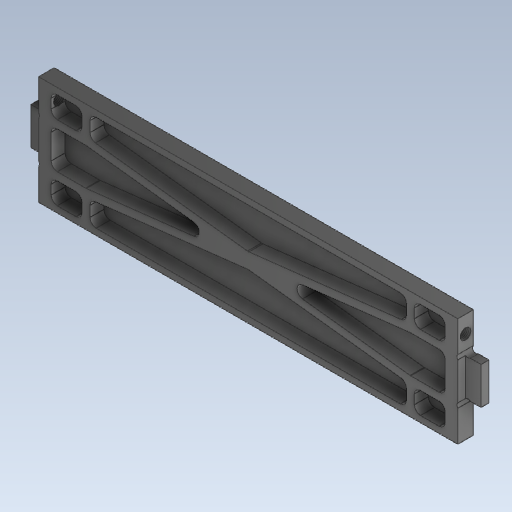
# Autodesk Inventor part: Cockpit_battery_front_frame
Saved by Autodesk Inventor 2020.4 (Build 244396000, 396)
## iProperties
Part Number: Cockpit_battery_front_frame
Material: アセタール樹脂、黒
Document SubType Name: Modeling
Designer: Masato Kubotera
Density: 1.425 g/cm^3
Appearance: 滑らか - 黒
Description: POM T5
Mass: 13.79 g
Surface Area: 149.623 cm^2
Volume: 9.6772 cm^3
Author: Masato Kubotera
Autodesk Inventor part; units mm, degrees
ref_plane "XZ Plane" through (0, 0, 0) normal (0, 1, 0) x (-1, 0, 0)
ref_plane "XY Plane" through (0, 0, 0) normal (0, 0, 1) x (1, 0, 0)
derived "Cockpit_side_frame.ipt"
sketch "スケッチ2" plane through (0, 0, 0) normal (0, 1, 0) x (-1, 0, 0)
  line L0 (-23.5, -22.5) -> (-28.5, -27.5)
  line L1 (-28.5, -27.5) -> (-28.5, -91)
  line L2 (-28.5, -91) -> (-23.5, -96)
  line L3 (-23.5, -96) -> (35.75, -96)
  line L4 (37.75, -98) -> (37.75, -131)
  line L5 (37.75, -131) -> (42.75, -136)
  line L6 (42.75, -136) -> (83.5, -136)
  line L7 (88.5, -131) -> (88.5, -20)
  line L8 (88.5, -20) -> (86, -17.5)
  line L9 (86, -17.5) -> (80.25, -17.5)
  line L10 (80.25, -17.5) -> (80.25, -21.0151)
  line L11 (78.7651, -22.5) -> (73.9849, -22.5)
  line L12 (72.5, -21.0151) -> (72.5, -17.5)
  line L13 (72.5, -17.5) -> (64.5, -17.5)
  line L14 (64.5, -17.5) -> (64.5, -21.0151)
  line L15 (63.0151, -22.5) -> (-23.5, -22.5)
  line L16 (-25.25, -25) -> (-20.25, -25) construction
  line L17 (-20.25, -25) -> (-20.25, -93.5) construction
  line L18 (-20.25, -93.5) -> (-25.25, -93.5) construction
  line L19 (-25.25, -93.5) -> (-25.25, -25) construction
  line L20 (-26, -25) -> (-25.25, -25) construction
  line L21 (-25.25, -93.5) -> (-26, -93.5) construction
  line L22 (-26, -93.5) -> (-26, -25) construction
  line L23 (-20.25, -93.5) -> (80.25, -93.5) construction
  line L24 (-20.25, -88.5) -> (80.25, -88.5) construction
  line L25 (80.25, -22.5) -> (80.25, -90.5) construction
  line L26 (80.25, -90.5) -> (85.25, -90.5) construction
  line L27 (85.25, -90.5) -> (85.25, -22.5) construction
  line L28 (80.25, -88.5) -> (80.25, -93.5) construction
  line L29 (80.25, -91) -> (85.25, -91) construction
  line L30 (85.25, -91) -> (85.25, -133.5) construction
  line L31 (80.25, -91) -> (80.25, -133.5) construction
  line L32 (80.25, -133.5) -> (85.25, -133.5) construction
  line L33 (40.25, -133.5) -> (40.25, -128.5) construction
  line L34 (40.25, -128.5) -> (40.25, -93.5) construction
  line L35 (45.25, -93.5) -> (45.25, -128.5) construction
  line L36 (40.25, -128.5) -> (45.25, -128.5) construction
  line L37 (42.75, -128.5) -> (42.75, -93.5) construction
  line L38 (40.25, -128.5) -> (79.1145, -128.5) construction
  line L39 (79.1145, -128.5) -> (79.1145, -133.5) construction
  line L40 (79.1145, -133.5) -> (40.25, -133.5) construction
  line L41 (40.25, -131) -> (79.1145, -131) construction
  line L42 (82.75, -91) -> (82.75, -133.5) construction
  circle A0 centre (82.75, -131) radius 2
  arc A1 (80.25, -128.5) -> (85.25, -128.5) centre (82.75, -131) ccw construction
  line L43 (80.25, -91) -> (-20.25, -91) construction
  line L44 (42.75, -111) -> (45.25, -111) construction
  line L45 (59.6822, -128.5) -> (59.6822, -131) construction
  line L46 (42.7, -115.5651) -> (42.7, -106.4349)
  line L47 (45.3, -107.05) -> (45.3, -114.95)
  line L48 (45.3, -117.05) -> (42.7, -104.95) construction
  line L49 (42.7, -117.05) -> (45.3, -104.95) construction
  line L50 (55.7322, -128.45) -> (63.6322, -128.45)
  line L51 (64.2473, -131.05) -> (55.1172, -131.05)
  line L52 (53.6322, -128.45) -> (65.7322, -131.05) construction
  line L53 (65.7322, -128.45) -> (53.6322, -131.05) construction
  line L54 (42.75, -105) -> (45.25, -105) construction
  line L55 (42.75, -117) -> (45.25, -117) construction
  arc A2 (44.1849, -104.95) -> (42.7, -106.4349) centre (43.4425, -105.6925) ccw
  arc A3 (45.3, -107.05) -> (45.3, -104.95) centre (45.3, -106) ccw
  arc A4 (42.7, -115.5651) -> (44.1849, -117.05) centre (43.4425, -116.3075) ccw
  arc A5 (45.3, -117.05) -> (45.3, -114.95) centre (45.3, -116) ccw
  line L56 (53.6822, -131) -> (53.6822, -128.5) construction
  line L57 (65.6822, -128.5) -> (65.6822, -131) construction
  arc A6 (53.6322, -129.5651) -> (55.1172, -131.05) centre (54.3747, -130.3075) ccw
  arc A7 (55.7322, -128.45) -> (53.6322, -128.45) centre (54.6822, -128.45) ccw
  arc A8 (64.2473, -131.05) -> (65.7322, -129.5651) centre (64.9898, -130.3075) ccw
  arc A9 (65.7322, -128.45) -> (63.6322, -128.45) centre (64.6822, -128.45) ccw
  line L58 (53.6322, -129.5651) -> (53.6322, -128.45)
  line L59 (65.7322, -128.45) -> (65.7322, -129.5651)
  line L60 (44.1849, -104.95) -> (45.3, -104.95)
  line L61 (45.3, -117.05) -> (44.1849, -117.05)
  circle A10 centre (47.6822, -131) radius 1.6
  line L62 (85.25, -22.5) -> (85.25, -17.5) construction
  line L63 (86, -17.5) -> (86, -90.5) construction
  line L64 (86, -90.5) -> (85.25, -90.5) construction
  line L65 (-18.5, -82.5) -> (-18.5, -61)
  arc A11 (-18.5, -82.5) -> (-16.5, -84.5) centre (-16.5, -82.5) ccw
  line L66 (45.5, -84.5) -> (-16.5, -84.5)
  arc A12 (45.5, -84.5) -> (47.5, -82.5) centre (45.5, -82.5) ccw
  line L67 (47.5, -61) -> (47.5, -82.5)
  arc A13 (47.5, -61) -> (45.5, -59) centre (45.5, -61) ccw
  line L68 (-16.5, -59) -> (45.5, -59)
  arc A14 (-16.5, -59) -> (-18.5, -61) centre (-16.5, -61) ccw
  line L69 (30, -88.5) -> (30, -91) construction
  line L70 (82.75, -22.5) -> (82.75, -90.5) construction
  circle A15 centre (82.75, -34) radius 1.6
  circle A16 centre (82.75, -34) radius 3
  circle A17 centre (82.75, -79) radius 3
  circle A18 centre (82.75, -79) radius 1.6
  line L71 (85.25, -22.5) -> (80.25, -22.5) construction
  arc A19 (85.25, -91) -> (80.25, -91) centre (82.75, -131) ccw construction
  circle A20 centre (47.6822, -131) radius 3
  circle A21 centre (42.75, -99) radius 1.6
  circle A22 centre (42.75, -99) radius 3
  line L72 (5, -88.5) -> (5, -91) construction
  line L73 (55, -88.5) -> (55, -91) construction
  line L74 (53.5651, -91.05) -> (6.4349, -91.05)
  line L75 (4.95, -89.5651) -> (4.95, -88.45)
  line L76 (7.05, -88.45) -> (52.95, -88.45)
  line L77 (55.05, -88.45) -> (55.05, -89.5651)
  line L78 (55.05, -91.05) -> (4.95, -88.45) construction
  line L79 (4.95, -91.05) -> (55.05, -88.45) construction
  arc A23 (7.05, -88.45) -> (4.95, -88.45) centre (6, -88.45) ccw
  arc A24 (4.95, -89.5651) -> (6.4349, -91.05) centre (5.6925, -90.3075) ccw
  arc A25 (53.5651, -91.05) -> (55.05, -89.5651) centre (54.3075, -90.3075) ccw
  arc A26 (55.05, -88.45) -> (52.95, -88.45) centre (54, -88.45) ccw
  line L80 (-20.25, -41) -> (80.25, -41) construction
  line L81 (80.25, -36) -> (-20.25, -36) construction
  line L82 (-20.25, -36) -> (-20.25, -41) construction
  line L83 (-20.25, -38.5) -> (80.25, -38.5) construction
  line L84 (30, -41) -> (30, -36) construction
  line L85 (53.5651, -35.95) -> (6.4349, -35.95)
  line L86 (6.4349, -41.05) -> (53.5651, -41.05)
  line L87 (55.05, -35.95) -> (4.95, -41.05) construction
  line L88 (4.95, -35.95) -> (55.5723, -41.1032) construction
  arc A27 (6.4349, -35.95) -> (4.95, -37.4349) centre (5.6925, -36.6925) ccw
  arc A28 (4.95, -39.5651) -> (6.4349, -41.05) centre (5.6925, -40.3075) ccw
  arc A29 (55.05, -37.4349) -> (53.5651, -35.95) centre (54.3075, -36.6925) ccw
  arc A30 (53.5651, -41.05) -> (55.05, -39.5651) centre (54.3075, -40.3075) ccw
  line L89 (5, -41) -> (5, -36) construction
  line L90 (55, -36) -> (55, -41) construction
  line L91 (4.95, -37.4349) -> (4.95, -39.5651)
  line L92 (55.05, -39.5651) -> (55.05, -37.4349)
  circle A31 centre (-2.5, -38.5) radius 1.6
  circle A32 centre (-2.5, -38.5) radius 3
  circle A33 centre (62.5, -38.5) radius 1.6
  circle A34 centre (62.5, -38.5) radius 3
  line L93 (-25.25, -44.25) -> (-22.75, -44.25) construction
  line L94 (-25.25, -49.25) -> (-26, -49.25) construction
  line L95 (-25.25, -74.25) -> (-22.75, -74.25) construction
  line L96 (-25.25, -69.25) -> (-26, -69.25) construction
  line L97 (-26, -59.25) -> (-25.25, -59.25) construction
  line L98 (-25.25, -59.25) -> (-22.75, -59.25) construction
  line L99 (-22.75, -25) -> (-22.75, -93.5) construction
  arc A35 (63.0151, -22.5) -> (64.5, -21.0151) centre (63.7575, -21.7575) ccw
  arc A36 (72.5, -21.0151) -> (73.9849, -22.5) centre (73.2425, -21.7575) ccw
  line L100 (56.75, -22.5) -> (56.75, -32.5) construction
  line L101 (56.75, -32.5) -> (80.25, -32.5) construction
  line L102 (80.25, -32.5) -> (80.25, -22.5) construction
  line L103 (68.5, -17.5) -> (68.5, -32.5) construction
  line L104 (60.5, -22.5) -> (60.5, -17.5) construction
  line L105 (76.5, -22.5) -> (76.5, -17.5) construction
  line L106 (-22.7, -46.3) -> (-22.7, -72.2)
  line L107 (-25.3, -72.8151) -> (-25.3, -69.564)
  line L108 (-25.3, -44.2) -> (-22.7, -74.3) construction
  line L109 (-22.7, -44.2) -> (-25.3, -74.3) construction
  arc A37 (-22.7, -46.3) -> (-22.7, -44.2) centre (-22.7, -45.25) ccw
  arc A38 (-23.8151, -44.2) -> (-25.3, -45.6849) centre (-24.5575, -44.9425) ccw
  line L110 (-23.8151, -44.2) -> (-22.7, -44.2)
  arc A39 (-25.3, -72.8151) -> (-23.8151, -74.3) centre (-24.5575, -73.5575) ccw
  arc A40 (-22.7, -74.3) -> (-22.7, -72.2) centre (-22.7, -73.25) ccw
  line L111 (-22.7, -74.3) -> (-23.8151, -74.3)
  line L112 (-26.3, -49.9848) -> (-26.3, -68.5152)
  arc A41 (-26.3, -68.5152) -> (-25.3, -69.564) centre (-25.25, -68.5152) ccw
  arc A42 (-25.3, -48.936) -> (-26.3, -49.9848) centre (-25.25, -49.9848) ccw
  line L113 (-25.3, -48.936) -> (-25.3, -45.6849)
  circle A43 centre (-22.75, -36.75) radius 1.6
  circle A44 centre (-22.75, -36.75) radius 3
  circle A45 centre (-22.75, -81.75) radius 1.6
  circle A46 centre (-22.75, -81.75) radius 3
  line L114 (64.5, -22.5) -> (72.5, -22.5)
  line L115 (85.25, -17.5) -> (52.5, -17.5) construction
  line L116 (52.5, -17.5) -> (52.5, -22.5) construction
  circle A47 centre (82.75, -93.5) radius 1.475
  circle A48 centre (82.75, -98.5) radius 1.475
  circle A49 centre (82.75, -103.5) radius 1.475
  line L117 (49.75, -93.5) -> (78.25, -93.5)
  line L118 (80.25, -95.5) -> (80.25, -124)
  line L119 (78.25, -126) -> (49.75, -126)
  line L120 (47.75, -124) -> (47.75, -95.5)
  arc A50 (49.75, -93.5) -> (47.75, -95.5) centre (49.75, -95.5) ccw
  arc A51 (47.75, -124) -> (49.75, -126) centre (49.75, -124) ccw
  arc A52 (78.25, -126) -> (80.25, -124) centre (78.25, -124) ccw
  arc A53 (80.25, -95.5) -> (78.25, -93.5) centre (78.25, -95.5) ccw
  arc A54 (37.75, -98) -> (35.75, -96) centre (35.75, -98) ccw
  circle A55 centre (-13.5, -55) radius 1.75
  circle A56 centre (-13.5, -55) radius 2
  line L121 (74.85, -78.65) -> (65.65, -78.65) construction
  line L122 (65.65, -78.65) -> (65.65, -64.85) construction
  line L123 (65.65, -64.85) -> (74.85, -64.85) construction
  line L124 (74.85, -64.85) -> (74.85, -78.65) construction
  line L125 (74.85, -78.65) -> (65.65, -64.85) construction
  line L126 (65.65, -78.65) -> (74.85, -64.85) construction
  line L127 (64.95, -64.2) -> (75.55, -64.2) construction
  line L128 (75.55, -64.2) -> (75.55, -79.3) construction
  line L129 (75.55, -79.3) -> (64.95, -79.3) construction
  line L130 (64.95, -79.3) -> (64.95, -64.2) construction
  line L131 (64.95, -64.2) -> (75.55, -79.3) construction
  line L132 (75.55, -64.2) -> (64.95, -79.3) construction
  line L133 (66.3849, -64.15) -> (74.1151, -64.15)
  line L134 (75.6, -65.6349) -> (75.6, -77.8651)
  line L135 (75.6, -79.35) -> (64.9, -64.15) construction
  line L136 (64.9, -79.35) -> (75.6, -64.15) construction
  line L137 (74.9, -78.7) -> (65.6, -64.8) construction
  line L138 (65.6, -78.7) -> (74.9, -64.8) construction
  arc A57 (66.3849, -64.15) -> (64.9, -65.6349) centre (65.6425, -64.8925) ccw
  arc A58 (67.0849, -64.8) -> (65.6, -66.2849) centre (66.3425, -65.5425) ccw
  line L139 (64.9, -71.75) -> (75.6, -71.75) construction
  line L140 (70.25, -64.15) -> (70.25, -78.7063) construction
  arc A59 (75.6, -65.6349) -> (74.1151, -64.15) centre (74.8575, -64.8925) ccw
  arc A60 (74.9, -66.2849) -> (73.4151, -64.8) centre (74.1575, -65.5425) ccw
  arc A61 (65.6, -77.2151) -> (67.0849, -78.7) centre (66.3425, -77.9575) ccw
  arc A62 (64.9, -77.8651) -> (66.3849, -79.35) centre (65.6425, -78.6075) ccw
  arc A63 (73.4151, -78.7) -> (74.9, -77.2151) centre (74.1575, -77.9575) ccw
  arc A64 (74.1151, -79.35) -> (75.6, -77.8651) centre (74.8575, -78.6075) ccw
  line L141 (67.0849, -64.8) -> (73.4151, -64.8)
  line L142 (74.9, -66.2849) -> (74.9, -77.2151)
  line L143 (64.9, -77.8651) -> (64.9, -65.6349)
  line L144 (65.6, -77.2151) -> (65.6, -66.2849)
  line L145 (73.4151, -78.7) -> (67.0849, -78.7)
  line L146 (74.1151, -79.35) -> (66.3849, -79.35)
  line L147 (-18.5, -71.75) -> (47.5, -71.75) construction
  line L148 (82.75, -56.5) -> (85.25, -56.5) construction
  line L149 (86, -54) -> (85.25, -54) construction
  line L150 (82.7, -69.45) -> (82.7, -43.55)
  line L151 (85.3057, -71.616) -> (82.7, -41.45) construction
  line L152 (82.7, -71.55) -> (85.3, -41.45) construction
  arc A65 (82.7, -41.45) -> (82.7, -43.55) centre (82.7, -42.5) ccw
  arc A66 (85.3, -42.9349) -> (83.8151, -41.45) centre (84.5575, -42.1925) ccw
  arc A67 (82.7, -69.45) -> (82.7, -71.55) centre (82.7, -70.5) ccw
  arc A68 (83.8151, -71.55) -> (85.3, -70.0651) centre (84.5575, -70.8075) ccw
  line L153 (82.75, -41.5) -> (85.25, -41.5) construction
  line L154 (82.75, -71.5) -> (85.25, -71.5) construction
  arc A69 (86.25, -47.1801) -> (85.3, -46.1348) centre (85.2, -47.1801) ccw
  line L155 (86.25, -47.1801) -> (86.25, -65.8199)
  line L156 (85.25, -46.5) -> (86, -46.5) construction
  line L157 (85.25, -66.5) -> (86, -66.5) construction
  arc A70 (85.3, -66.8652) -> (86.25, -65.8199) centre (85.2, -65.8199) ccw
  line L158 (85.3, -42.9349) -> (85.3, -46.1348)
  line L159 (85.3, -66.8652) -> (85.3, -70.0651)
  line L160 (83.8151, -71.55) -> (82.7, -71.55)
  line L161 (82.7, -41.45) -> (83.8151, -41.45)
  line L162 (83.5, -136) -> (88.5, -131)
  arc A71 (78.7651, -22.5) -> (80.25, -21.0151) centre (79.5075, -21.7575) ccw
  point P0 (0, 0)
  point P1 (-25.7227, -96)
  point P2 (-23.5, -22.5)
  point P3 (44, -111)
  point P4 (59.6822, -129.75)
  point P5 (30, -89.75)
  point P6 (30, -38.5)
  point P7 (4.95, -41.05)
  point P8 (52.5, -22)
  point P9 (-24, -59.25)
  point P10 (70.25, -71.75)
  point P11 (70.25, -71.75)
  point P12 (84, -56.5)
  point P13 (80.25, -22.5)
  dimension "d1" = 45.25
  dimension "d2" = 5
  dimension "d3" = 2.5
  measures "d1" distance from line of point (0, 0) L35
  measures "d2" distance of L35.end L33.end
  measures "d3" distance of L55.start L55.end
ref_plane "作業平面1" through (-45.25, 0, 0) normal (1, 0, 0) x (0, 1, 0)
sketch "スケッチ3" plane through (-45.25, 0, 0) normal (1, 0, 0) x (0, 1, 0)
  line L0 (-135, -93.5) -> (0, -93.5)
  line L1 (0, -128.5) -> (-135, -128.5)
  line L2 (1.4849, -105) -> (5, -105)
  line L3 (5, -105) -> (5, -117)
  arc A0 (0, -103.5151) -> (1.4849, -105) centre (0.7425, -104.2575) ccw
  line L4 (0, -93.5) -> (0, -103.5151)
  line L5 (-134.9908, -111) -> (0, -111) construction
  line L6 (1.4849, -117) -> (5, -117)
  arc A1 (1.4849, -117) -> (0, -118.4849) centre (0.7425, -117.7425) ccw
  line L7 (0, -128.5) -> (0, -118.4849)
  line L8 (0, -105) -> (0, -117)
  line L9 (0, -118.4849) -> (0, -128.5)
  line L10 (-67.5, -93.5) -> (-67.5, -128.5) construction
  line L11 (-136.4849, -105) -> (-140, -105)
  line L12 (-140, -105) -> (-140, -117)
  arc A2 (-136.4849, -105) -> (-135, -103.5151) centre (-135.7425, -104.2575) ccw
  line L13 (-135, -93.5) -> (-135, -103.5151)
  line L14 (-136.4849, -117) -> (-140, -117)
  arc A3 (-135, -118.4849) -> (-136.4849, -117) centre (-135.7425, -117.7425) ccw
  line L15 (-135, -128.5) -> (-135, -118.4849)
  line L16 (-135, -105) -> (-135, -117)
  line L17 (-135, -118.4849) -> (-135, -128.5)
  line L18 (-12, -119.5) -> (-6, -119.5)
  line L19 (-4, -121.5) -> (-4, -124.5)
  line L20 (-6, -126.5) -> (-12, -126.5)
  line L21 (-14, -124.5) -> (-14, -121.5)
  line L22 (-4, -115) -> (-4, -107)
  line L23 (-67.2707, -113.5132) -> (-18.2707, -119.168)
  line L24 (-16.5, -121.1548) -> (-16.5, -124.5)
  line L25 (-18.5, -126.5) -> (-116.5, -126.5)
  line L26 (-6, -117) -> (-15.135, -117)
  line L27 (-15.3643, -116.9868) -> (-50.0251, -112.9868)
  line L28 (-12, -102.5) -> (-6, -102.5)
  line L29 (-4, -100.5) -> (-4, -97.5)
  line L30 (-6, -95.5) -> (-12, -95.5)
  line L31 (-14, -97.5) -> (-14, -100.5)
  line L32 (-67.2707, -108.4868) -> (-18.2707, -102.832)
  line L33 (-16.5, -100.8452) -> (-16.5, -97.5)
  line L34 (-18.5, -95.5) -> (-116.5, -95.5)
  line L35 (-6, -105) -> (-15.135, -105)
  line L36 (-15.3643, -105.0132) -> (-50.0251, -109.0132)
  line L37 (-67.7293, -113.5132) -> (-116.7293, -119.168)
  line L38 (-118.5, -121.1548) -> (-118.5, -124.5)
  line L39 (-118.5, -100.8452) -> (-118.5, -97.5)
  line L40 (-67.7293, -108.4868) -> (-116.7293, -102.832)
  arc A4 (-6, -126.5) -> (-4, -124.5) centre (-6, -124.5) ccw
  arc A5 (-4, -121.5) -> (-6, -119.5) centre (-6, -121.5) ccw
  arc A6 (-12, -119.5) -> (-14, -121.5) centre (-12, -121.5) ccw
  arc A7 (-14, -124.5) -> (-12, -126.5) centre (-12, -124.5) ccw
  arc A8 (-18.5, -126.5) -> (-16.5, -124.5) centre (-18.5, -124.5) ccw
  arc A9 (-16.5, -121.1548) -> (-18.2707, -119.168) centre (-18.5, -121.1548) ccw
  arc A10 (-67.2707, -113.5132) -> (-67.7293, -113.5132) centre (-67.5, -115.5) ccw
  arc A11 (-116.7293, -119.168) -> (-118.5, -121.1548) centre (-116.5, -121.1548) ccw
  arc A12 (-118.5, -124.5) -> (-116.5, -126.5) centre (-116.5, -124.5) ccw
  arc A13 (-118.5, -100.8452) -> (-116.7293, -102.832) centre (-116.5, -100.8452) ccw
  arc A14 (-116.5, -95.5) -> (-118.5, -97.5) centre (-116.5, -97.5) ccw
  arc A15 (-16.5, -97.5) -> (-18.5, -95.5) centre (-18.5, -97.5) ccw
  arc A16 (-18.2707, -102.832) -> (-16.5, -100.8452) centre (-18.5, -100.8452) ccw
  arc A17 (-67.7293, -108.4868) -> (-67.2707, -108.4868) centre (-67.5, -106.5) ccw
  arc A18 (-50.0251, -109.0132) -> (-50.0251, -112.9868) centre (-49.7958, -111) ccw
  arc A19 (-15.135, -105) -> (-15.3643, -105.0132) centre (-15.135, -107) ccw
  arc A20 (-4, -107) -> (-6, -105) centre (-6, -107) ccw
  arc A21 (-6, -117) -> (-4, -115) centre (-6, -115) ccw
  arc A22 (-15.3643, -116.9868) -> (-15.135, -117) centre (-15.135, -115) ccw
  arc A23 (-14, -100.5) -> (-12, -102.5) centre (-12, -100.5) ccw
  arc A24 (-12, -95.5) -> (-14, -97.5) centre (-12, -97.5) ccw
  arc A25 (-4, -97.5) -> (-6, -95.5) centre (-6, -97.5) ccw
  arc A26 (-6, -102.5) -> (-4, -100.5) centre (-6, -100.5) ccw
  line L41 (-123, -119.5) -> (-129, -119.5)
  line L42 (-121, -124.5) -> (-121, -121.5)
  line L43 (-131, -115) -> (-131, -107)
  line L44 (-129, -117) -> (-119.865, -117)
  line L45 (-119.6357, -116.9868) -> (-84.9749, -112.9868)
  line L46 (-123, -102.5) -> (-129, -102.5)
  line L47 (-121, -97.5) -> (-121, -100.5)
  line L48 (-129, -95.5) -> (-123, -95.5)
  line L49 (-131, -100.5) -> (-131, -97.5)
  line L50 (-119.6357, -105.0132) -> (-84.9749, -109.0132)
  line L51 (-129, -105) -> (-119.865, -105)
  arc A27 (-131, -124.5) -> (-129, -126.5) centre (-129, -124.5) ccw
  arc A28 (-129, -119.5) -> (-131, -121.5) centre (-129, -121.5) ccw
  arc A29 (-121, -121.5) -> (-123, -119.5) centre (-123, -121.5) ccw
  arc A30 (-123, -126.5) -> (-121, -124.5) centre (-123, -124.5) ccw
  arc A31 (-84.9749, -112.9868) -> (-84.9749, -109.0132) centre (-85.2042, -111) ccw
  arc A32 (-119.6357, -105.0132) -> (-119.865, -105) centre (-119.865, -107) ccw
  arc A33 (-129, -105) -> (-131, -107) centre (-129, -107) ccw
  arc A34 (-131, -115) -> (-129, -117) centre (-129, -115) ccw
  arc A35 (-119.865, -117) -> (-119.6357, -116.9868) centre (-119.865, -115) ccw
  arc A36 (-123, -102.5) -> (-121, -100.5) centre (-123, -100.5) ccw
  arc A37 (-121, -97.5) -> (-123, -95.5) centre (-123, -97.5) ccw
  arc A38 (-129, -95.5) -> (-131, -97.5) centre (-129, -97.5) ccw
  arc A39 (-131, -100.5) -> (-129, -102.5) centre (-129, -100.5) ccw
  line L52 (-129, -126.5) -> (-123, -126.5)
  line L53 (-4, -99) -> (0, -99) construction
  line L54 (-131, -121.5) -> (-131, -124.5)
  point P0 (0, 0)
  point P1 (0, -128.5)
  point P2 (-135, -111)
  point P3 (-14, -119.5)
  point P4 (-4, -126.5)
  point P5 (-4, -119.5)
  point P6 (-14, -126.5)
  point P7 (-4, -117)
  point P8 (-67.5, -113.4867)
  point P9 (-16.5, -119.3723)
  point P10 (-16.5, -126.5)
  point P11 (-118.5, -126.5)
  point P12 (-15.25, -117)
  point P13 (-67.2412, -111)
  point P14 (-14, -102.5)
  point P15 (-4, -95.5)
  point P16 (-4, -102.5)
  point P17 (-14, -95.5)
  point P18 (-4, -105)
  point P19 (-67.5, -108.5133)
  point P20 (-16.5, -102.6277)
  point P21 (-16.5, -95.5)
  point P22 (-15.25, -105)
  point P23 (-118.5, -119.3723)
  point P24 (-118.5, -126.5)
  point P25 (-118.5, -102.6277)
  point P26 (-118.5, -95.5)
  dimension "d5" = 5
  dimension "d6" = 135
  dimension "d7" = 1.05
  dimension "d19" = 4
  dimension "d20" = 2
  dimension "d21" = 10
  dimension "d22" = 2.5
  dimension "d23" = 11.25
  dimension "d24" = 2.5
  dimension "d25" = 2
  dimension "d26" = 2.5
  dimension "d27" = 5
  constraints: 110 end point, 85 point on circle, 72 symmetric about line, 58 point on line, 46 tangent, 40 centre point, 22 equal radius, 9 perpendicular, 5 midpoint, 5 parallel, 4 horizontal, 3 coincident, 2 collinear, 1 vertical, 16 other
  measures "d5" distance between parallel lines of L3 L8
  measures "d6" distance of L0.start L0.end
  measures "d7" radius of A0
  measures "d19" distance between parallel lines of L7 L19
  measures "d20" distance between parallel lines of L1 L20
  measures "d21" distance of point (-4, -126.5) point (-14, -126.5)
  measures "d22" distance between parallel lines of L24 L21
  measures "d23" distance of point (-4, -117) point (-15.25, -117)
  measures "d24" distance between parallel lines of L23 L27
  measures "d25" radius of A4
  measures "d26" distance between parallel lines of L18 L26
extrude "押し出し1" add sketch "スケッチ3" along normal blind 5 contours L0 L4 A0 L8 A1 L7 L1 L15 A3 L16 A2 L13
extrude "押し出し2" add sketch "スケッチ3" along normal blind 2.5 contours L16 A3 L14 L12 L11 A2 | A0 L2 L3 L6 A1 L8
hole "穴1" at (-42.75, 0, -99) direction (0, -1, 0) diameter 3.4587 depth 4 thread size "M4x0.5" class "6H" standard "ANSI Metric M Profile"
ref_plane "作業平面2" through (-45.25, -67.5, -93.5) normal (0, 1, 0) x (1, 0, 0)
mirror "ミラー1" about plane through (-45.25, -67.5, -93.5) normal (0, 1, 0) of "穴1"
extrude "押し出し3" add sketch "スケッチ3" along normal blind 0.5 contours L18 A5 L19 A4 L20 A7 L21 A6 | A21 L26 A22 L27 A18 L36 A19 L35 A20 L22 | L23 A9 L24 A8 L25 A12 L38 A11 L37 A10 | A23 L31 A24 L30 A25 L29 A26 L28 | A17 L40 A13 L39 A14 L34 A15 L33 A16 L32 | A29 L42 A30 L52 A27 L54 A28 L41 | L43 A33 L51 A32 L50 A31 L45 A35 L44 A34 | L46 A39 L49 A38 L48 A37 L47 A36
equation "\"d23\" = d21 + 0.5 * d22"
equation "\"d24\" = d22"
equation "\"d26\" = d22"
equation "\"d27\" = 2 * d22"
equation "\"d8\" = d2"
equation "\"d10\" = d3"
equation "\"d4\" = -d1"
